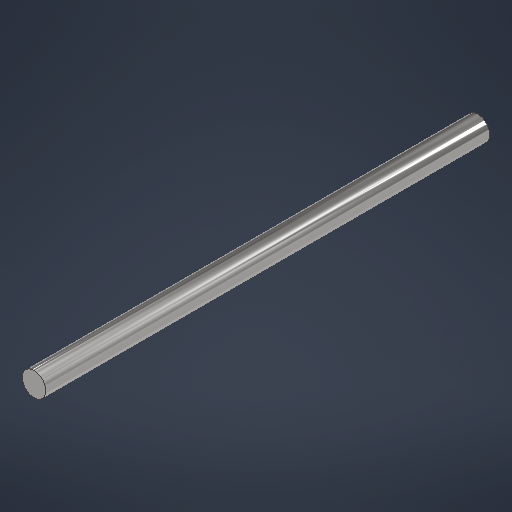
# Autodesk Inventor part: M3 Pivot Rod
Saved by Autodesk Inventor 2026.1 (Build 301233020, 233B)
## iProperties
Created: 2026-04-17
Part Number: M3 Pivot Rod
Material: Generic
Document SubType Name: Modeling
Designer: Bahaa
Mass: 0.399375 g
Surface Area: 5.46637 cm^2
Volume: 0.399375 cm^3
Density: 1 g/cm^3
Appearance: Steel - Polished
Author: Bahaa
Autodesk Inventor part; units mm, degrees
ref_plane "YZ Plane" through (0, 0, 0) normal (1, 0, 0) x (0, 1, 0)
ref_plane "XZ Plane" through (0, 0, 0) normal (0, 1, 0) x (-1, 0, 0)
ref_plane "XY Plane" through (0, 0, 0) normal (0, 0, 1) x (1, 0, 0)
sketch "Sketch1" plane through (0, 0, 0) normal (0, 1, 0) x (-1, 0, 0)
  circle A0 centre (0, 0) radius 1.5
  dimension "d0" = 3
  constraints: 1 centre point, 1 coincident
  measures "d0" diameter of A0
extrude "Extrusion1" add sketch "Sketch1" along normal blind 56.5
body "Solid1"
